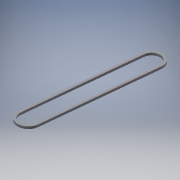
# Autodesk Inventor part: ketting2
Saved by Autodesk Inventor 2017 (Build 210142000, 142)
## iProperties
Created: 2017-02-19
Part Number: ketting2
Material: Generic
Document SubType Name: Modeling
Designer: user
Density: 1 g/cm^3
Appearance: Default
Author: user
Autodesk Inventor part; units mm, degrees
ref_plane "YZ Plane" through (0, 0, 0) normal (1, 0, 0) x (0, 1, 0)
ref_plane "XZ Plane" through (0, 0, 0) normal (0, 1, 0) x (-1, 0, 0)
ref_plane "XY Plane" through (0, 0, 0) normal (0, 0, 1) x (1, 0, 0)
sketch "Sketch1" plane through (0, 0, 0) normal (0, 0, 1) x (1, 0, 0)
  circle A0 centre (-138.7819, 17.9715) radius 30 projected
  circle A1 centre (-40, -365) radius 10 projected
  circle A2 centre (-40, -365) radius 30 projected
  line L0 (-76.7957, -374.4909) -> (-175.5776, 8.4805)
  arc A3 (-101.9862, 27.4624) -> (-175.5776, 8.4805) centre (-138.7819, 17.9715) ccw
  line L1 (-101.9862, 27.4624) -> (-3.2043, -355.5091)
  arc A4 (-76.7957, -374.4909) -> (-3.2043, -355.5091) centre (-40, -365) ccw
  line L2 (-10.9508, -357.5072) -> (-109.7327, 25.4643)
  arc A5 (-109.7327, 25.4643) -> (-167.8311, 10.4786) centre (-138.7819, 17.9715) ccw
  line L3 (-167.8311, 10.4786) -> (-69.0492, -372.4928)
  arc A6 (-69.0492, -372.4928) -> (-10.9508, -357.5072) centre (-40, -365) ccw
  point P0 (0, 0)
  dimension "d0" = 8
  constraints: 8 end point, 8 point on circle, 5 tangent, 4 centre point, 2 concentric, 2 parallel, 3 other
  measures "d0" distance between parallel lines of L1 L2
extrude "Extrusion1" add sketch "Sketch1" against normal blind 8 contours L0 A3 L1 A4
body "Solid1"
